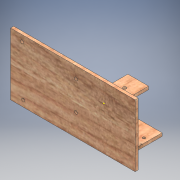
# Autodesk Inventor part: podstawa
Saved by Autodesk Inventor 2017 (Build 210142000, 142)
## iProperties
Created: 2017-05-15
Part Number: podstawa
Material: Drewno (brzoza)
Document SubType Name: Modeling
Designer: Damian
Density: 0.55 g/cm^3
Appearance: Brzoza — naturalna — polerowana
Author: Damian
Autodesk Inventor part; units mm, degrees
ref_plane "YZ Plane" through (0, 0, 0) normal (1, 0, 0) x (0, 1, 0)
ref_plane "XZ Plane" through (0, 0, 0) normal (0, 1, 0) x (-1, 0, 0)
ref_plane "XY Plane" through (0, 0, 0) normal (0, 0, 1) x (1, 0, 0)
sketch "Szkic1" plane through (0, 0, 0) normal (0, 1, 0) x (-1, 0, 0)
  line L0 (30, -30) -> (-30, -30)
  line L1 (-30, -30) -> (-30, 30)
  line L2 (-30, 30) -> (30, 30)
  line L3 (30, 30) -> (30, -30)
  line L4 (30, -30) -> (-30, 30) construction
  line L5 (-30, -30) -> (30, 30) construction
  point P0 (0, 0)
  dimension "d0" = 60
  dimension "d1" = 60
  constraints: 12 end point, 2 midpoint, 2 parallel, 1 horizontal, 1 perpendicular
  measures "d0" distance of L0.start L0.end
  measures "d1" distance of L0.end L1.end
extrude "Wyciągnięcie proste1" add sketch "Szkic1" along normal blind 3
sketch "Szkic2" plane through (0, 3, 0) normal (0, 1, 0) x (1, 0, 0)
  line L0 (10, -12) -> (-10, -12)
  line L1 (-10, -12) -> (-10, -15)
  line L2 (-10, -15) -> (10, -15)
  line L3 (10, -15) -> (10, -12)
  point P0 (0, 0)
  dimension "d4" = 20
  dimension "d5" = 3
  dimension "d6" = 12
  dimension "d7" = 10
  constraints: 8 end point, 2 parallel, 1 horizontal, 1 perpendicular
  measures "d4" distance of L2.end L1.end
  measures "d5" distance of L1.end L0.end
  measures "d6" distance from line of L0 point (0, 0)
  measures "d7" distance from line of point (0, 0) L1
sketch "Szkic3" plane through (0, 3, 0) normal (0, 1, 0) x (1, 0, 0)
  point P0 (0, 0)
sketch "Szkic4" plane through (0, 3, 0) normal (0, 1, 0) x (1, 0, 0)
  line L0 (-13, 17.5) -> (23, 17.5)
  line L1 (23, 17.5) -> (23, 20.5)
  line L2 (23, 20.5) -> (-13, 20.5)
  line L3 (-13, 20.5) -> (-13, 17.5)
  point P0 (0, 0)
  dimension "d8" = 3
  dimension "d9" = 36
  dimension "d10" = 17.5
  dimension "d11" = 13
  constraints: 8 end point, 2 parallel, 1 horizontal, 1 perpendicular
  measures "d8" distance of L0.end L1.end
  measures "d9" distance of L1.end L2.end
  measures "d10" distance from line of point (0, 0) L0
  measures "d11" distance from line of point (0, 0) L3
extrude "Wyciągnięcie proste2" add sketch "Szkic4" along normal blind 30
sketch "Szkic5" plane through (23, 3, -20.5) normal (0, 0, -1) x (-1, 0, 0)
  line L0 (0, 30) -> (36, 30) projected
  line L1 (36, 0) -> (36, 30) projected
  arc A0 (17.4615, 14.6923) -> (17.4615, 19.3077) centre (23, 17) ccw
  arc A1 (17.4615, 19.3077) -> (17.4615, 14.6923) centre (16.5, 17) ccw
  line L2 (0, 0) -> (0, 30) projected
  circle A2 centre (4.5, 17) radius 1.25
  circle A3 centre (31.5, 17) radius 1.25
  point P0 (23, -3)
  dimension "d14" = 13
  dimension "d15" = 13
  dimension "d16" = 12
  dimension "d17" = 6.5
  dimension "d18" = 5
  dimension "d19" = 4.5
  dimension "d20" = 4.5
  dimension "d21" = 2.5
  dimension "d22" = 2.5
  constraints: 4 centre point, 4 coincident, 4 point on circle
  measures "d14" distance from line of L0 point (23, 17)
  measures "d15" distance from line of L1 point (23, 17)
  measures "d16" diameter of A0
  measures "d17" distance of A0.centre point (16.5, 17)
  measures "d18" diameter of A1
  measures "d19" distance from line of L1 point (31.5, 17)
  measures "d20" distance from line of L2 point (4.5, 17)
  measures "d21" diameter of A2
  measures "d22" diameter of A3
extrude "Wyciągnięcie proste3" cut sketch "Szkic5" against normal blind 30
sketch "Szkic6" plane through (0, 3, 0) normal (0, 1, 0) x (1, 0, 0)
  point P0 (0, 0)
extrude "Wyciągnięcie proste4" add sketch "Szkic2" along normal blind 30
sketch "Szkic7" plane through (10, 3, 12) normal (0, 0, -1) x (-1, 0, 0)
  point P0 (10, -3)
sketch "Szkic8" plane through (-10, 3, 15) normal (0, 0, 1) x (1, 0, 0)
  line L0 (20, 0) -> (0, 0) projected
  point P0 (10, -3)
  point P1 (10, 17)
  dimension "d27" = 17
  measures "d27" distance from line of L0 point (10, 17)
hole "Otwór1" at (0, 20, 15) direction (0, 0, -1) diameter 3.2 end through all
sketch "Szkic9" plane through (-30, 0, -30) normal (-1, 0, 0) x (0, 0, 1)
  line L0 (60, 3) -> (0, 3) projected
  line L1 (0, 0) -> (60, 0)
  line L2 (60, 0) -> (60, 3)
  line L3 (60, 3) -> (0, 3)
  line L4 (0, 3) -> (0, 0)
  point P0 (30, 0)
  constraints: 8 end point, 2 parallel, 1 horizontal, 1 perpendicular
extrude "Wyciągnięcie proste5" add sketch "Szkic9" along normal blind 60
sketch "Szkic10" plane through (0, 3, 0) normal (0, 1, 0) x (1, 0, 0)
  line L0 (-13, 20.5) -> (-13, 17.5) projected
  line L1 (30, -30) -> (-90, -30) projected
  point P0 (0, 0)
  point P1 (-27, -19)
  point P2 (-27, 8.9)
  point P3 (-77.8, 24)
  point P4 (-79.1, -24.1)
  dimension "d38" = 14
  dimension "d39" = 11
  dimension "d40" = 27.9
  dimension "d41" = 50.8
  dimension "d42" = 54
  dimension "d43" = 1.3
  dimension "d44" = 5.9
  measures "d38" distance from line of L0 point (-27, -19)
  measures "d39" distance from line of L1 point (-27, -19)
  measures "d40" distance of point (-27, -19) point (-27, 8.9)
  measures "d41" horizontal distance of point (-77.8, 24) point (-27, 8.9)
  measures "d42" distance from line of L1 point (-77.8, 24)
  measures "d43" horizontal distance of point (-79.1, -24.1) point (-77.8, 24)
  measures "d44" distance from line of L1 point (-79.1, -24.1)
hole "Otwór2" at (-27, 3, 19) at (-27, 3, -8.9) at (-77.8, 3, -24) at (-79.1, 3, 24.1) direction (0, -1, 0) diameter 3 end through all
